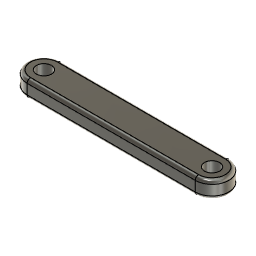
Camera Stand Part 2 (Autodesk Fusion 360 design; units mm, degrees)
Autodesk Fusion 360 part; units mm, degrees
sketch "Sketch1" plane through (0, 0, 0) normal (0, 0, 1) x (1, 0, 0)
  line L0 (-25, 5) -> (25, 5)
  line L1 (25, 5) -> (25, -5)
  line L2 (25, -5) -> (-25, -5)
  line L3 (-25, -5) -> (-25, 5)
  line L4 (-25, 5) -> (25, -5) construction
  line L5 (25, 5) -> (-25, -5) construction
  dimension "d1" = 50
  dimension "d2" = 10
  constraint horizontal L0
  constraint perpendicular L0 L1
  constraint parallel L0 L2
  constraint parallel L1 L3
  constraint coincident L4 origin
  constraint coincident L5 origin
  measures "d1" distance of L1.end L2.end
  measures "d2" distance of L0.end L1.end
sketch "Sketch2" plane through (0, 0, 0) normal (0, 0, 1) x (1, 0, 0)
  line L0 (0, 0) -> (25, 0)
  circle A0 centre (25, 0) radius 5
  line L1 (0, 0) -> (-25, 0)
  circle A1 centre (-25, 0) radius 5
  dimension "d3" = 25
  dimension "d4" = 10
  dimension "d5" = 25
  dimension "d6" = 10
  constraint coincident L0.start L1.start
  constraint horizontal L0
  constraint coincident L0.end A0.centre
  constraint parallel L0 L1
  constraint coincident L1.end A1.centre
  measures "d3" distance of L0.start L0.end
  measures "d4" diameter of A0
  measures "d5" distance of L0.start L1.end
  measures "d6" diameter of A1
extrude "Extrude1" add sketch "Sketch2" sketch "Sketch1" along normal blind 5 of sketch 2
hole "Hole1" at (25, 0, 5) direction (0, 0, -1) diameter 4.5 depth 5 tip angle 118
hole "Hole2" at (-25, 0, 5) direction (0, 0, -1) diameter 4.5 depth 5 tip angle 118
fillet "Fillet3" radius 1 4 edges at (30, 0, 5) (0, 5, 5) (-30, 0, 5) (0, -5, 5)
fillet "Fillet4" radius 1 4 edges at (0, -5, 0) (30, 0, 0) (0, 5, 0) (-30, 0, 0)
sketch "Sketch3" plane through (0, 0, 5) normal (0, 0, 1) x (-1, 0, 0)
  arc A0 (-25, 5) -> (-25, -5) centre (-25, 0) ccw
  line L0 (-25, -5) -> (25, -5)
  arc A1 (25, -5) -> (25, 5) centre (25, 0) ccw
  line L1 (25, 5) -> (-25, 5)
  circle A2 centre (-25, 0) radius 2
  circle A3 centre (25, 0) radius 2
  dimension "d9" = 4
  dimension "d10" = 4
  constraint concentric A0 A2
  constraint concentric A1 A3
  measures "d9" diameter of A2
  measures "d10" diameter of A3
extrude "Extrude2" [suppressed]
fillet "Fillet1" [suppressed]
fillet "Fillet2" [suppressed]
